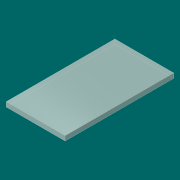
# Autodesk Inventor part: bottom
Saved by Autodesk Inventor 2016 (Build 200138000, 138)
## iProperties
Created: 2015-10-13
Part Number: bottom
Material: PC/ABS Plastic
Document SubType Name: Modeling
Designer: Sawaiz
Density: 0.357273 g/cm^3
Appearance: Clear
Author: Sawaiz
Autodesk Inventor part; units mm, degrees
ref_plane "YZ Plane" through (0, 0, 0) normal (1, 0, 0) x (0, 1, 0)
ref_plane "XZ Plane" through (0, 0, 0) normal (0, 1, 0) x (-1, 0, 0)
ref_plane "XY Plane" through (0, 0, 0) normal (0, 0, 1) x (1, 0, 0)
sketch "Sketch1" plane through (0, 0, 0) normal (0, 0, 1) x (1, 0, 0)
  line L0 (-111.125, -60.325) -> (111.125, -60.325)
  line L1 (111.125, -60.325) -> (111.125, 60.325)
  line L2 (111.125, 60.325) -> (-111.125, 60.325)
  line L3 (-111.125, 60.325) -> (-111.125, -60.325)
  line L4 (-111.125, -60.325) -> (111.125, 60.325) construction
  line L5 (111.125, -60.325) -> (-111.125, 60.325) construction
  point P0 (0, 0)
  dimension "d0" = 222.25
  dimension "d1" = 120.65
  constraints: 12 end point, 2 midpoint, 2 parallel, 1 horizontal, 1 perpendicular
  measures "d0" distance of L2.end L1.end
  measures "d1" distance of L1.end L0.end
extrude "Extrusion1" add sketch "Sketch1" along normal blind 9.525
equation "\"d0\" = depth + 2 * frameAcrylicThickness"
equation "\"d1\" = width + 2 * frameAcrylicThickness"
equation "\"d2\" = frameAcrylicThickness"
equation "\"width\" = 101.6"
equation "\"depth\" = 203.2"
equation "\"fresnelThickness\" = 0.1"
equation "\"centerThickness\" = 1.524"
equation "\"frameAcrylicThickness\" = 9.525"
equation "\"internalAcrylicThickness\" = 6.35"
equation "\"aerogelWidth\" = 101.6"
equation "\"aerogelHeight\" = 101.6"
equation "\"height\" = 101.6"
equation "\"mirrorAngle\" = 5deg"
equation "\"detectorWidth\" = 52"
equation "\"detectorHeight\" = 52"
equation "\"mirrorThickness\" = 3.175"
equation "\"focalLength\" = 76.2"
equation "\"ior\" = 1.49"
equation "\"fresnelAngle\" = 90deg"
equation "\"fresnelEffectiveDiameter\" = 76.2"
equation "\"oRingWidth\" = 1.5875"
equation "\"sensorHolderDepth\" = 19.05"
body "Solid1"
